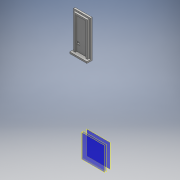
# Autodesk Inventor part: goraczesc1zotworem
Saved by Autodesk Inventor 2016 SP1 (Build 200210100, 210)
## iProperties
Created: 2019-02-21
Part Number: goraczesc1zotworem
Material: Ogólny
Document SubType Name: Modeling
Designer: Maciek
Density: 1 g/cm^3
Appearance: Domyślna
Author: Maciek
Autodesk Inventor part; units mm, degrees
ref_plane "YZ Plane" through (0, 0, 0) normal (1, 0, 0) x (0, 1, 0)
ref_plane "XZ Plane" through (0, 0, 0) normal (0, 1, 0) x (-1, 0, 0)
ref_plane "XY Plane" through (0, 0, 0) normal (0, 0, 1) x (1, 0, 0)
ref_plane "Płaszczyzna konstrukcyjna1" through (0, 19, 0) normal (0, 1, 0) x (1, 0, 0)
ref_plane "Płaszczyzna konstrukcyjna3" through (0, 19, 0) normal (0, 1, 0) x (1, 0, 0)
ref_plane "Płaszczyzna konstrukcyjna2" through (0, 24, 0) normal (0, 1, 0) x (1, 0, 0)
sketch "Szkic23" plane through (0, 24, 0) normal (0, 1, 0) x (1, 0, 0)
  line L0 (-21.8, -101.1) -> (-21.8, -97.6) projected
  line L1 (-8.8, -67.6) -> (-8.8, -69.1) projected
  line L2 (-21.8, -101.1) -> (-8.8, -101.1)
  line L3 (-8.8, -101.1) -> (-8.8, -69.1)
  line L4 (-8.8, -69.1) -> (-21.8, -69.1)
  line L5 (-21.8, -69.1) -> (-21.8, -101.1)
  line L6 (-21.8, -101.1) -> (-20.3, -101.1) construction
  line L7 (-20.3, -101.1) -> (-20.3, -99.6) construction
  line L8 (-20.3, -99.6) -> (-21.8, -99.6) construction
  line L9 (-21.8, -99.6) -> (-21.8, -101.1) construction
  line L10 (-8.8, -69.1) -> (-10.3, -69.1) construction
  line L11 (-21.8, -69.1) -> (-8.8, -69.1) construction
  line L12 (-20.3, -99.6) -> (-10.3, -99.6)
  line L13 (-10.3, -99.6) -> (-10.3, -69.1)
  line L14 (-10.3, -69.1) -> (-20.3, -69.1)
  line L15 (-20.3, -69.1) -> (-20.3, -99.6)
  point P0 (0, 0)
  dimension "d135" = 1.5
  dimension "d136" = 1.5
  dimension "d137" = 1.5
  constraints: 26 end point, 6 parallel, 3 horizontal, 3 perpendicular, 1 point on line
  measures "d135" distance of L8.end L7.end
  measures "d136" distance of L7.end L6.end
  measures "d137" distance of L1.end L10.end
extrude "Wyciągnięcie proste21" add sketch "Szkic23" against normal blind 1.5 contours L0 L5 L4 L15 L12 L13 L3 L2
ref_plane "Płaszczyzna konstrukcyjna5" through (0, 24, 0) normal (0, 1, 0) x (1, 0, 0)
sketch "Szkic24" plane through (0, 24, 0) normal (0, 1, 0) x (1, 0, 0)
  line L0 (-23.3, -69.1) -> (-23.3, -102.6) projected
  line L1 (-23.3, -69.1) -> (-7.3, -69.1)
  line L2 (-7.3, -69.1) -> (-7.3, -67.6)
  line L3 (-7.3, -67.6) -> (-23.3, -67.6)
  line L4 (-23.3, -67.6) -> (-23.3, -69.1)
  point P0 (0, 0)
  dimension "d140" = 16
  dimension "d141" = 1.5
  constraints: 8 end point, 2 parallel, 1 horizontal, 1 perpendicular
  measures "d140" distance of L3.end L2.end
  measures "d141" distance of L2.end L1.end
extrude "Wyciągnięcie proste22" add sketch "Szkic24" against normal blind 3.5
ref_plane "Płaszczyzna konstrukcyjna6" through (0, 24, 0) normal (0, 1, 0) x (1, 0, 0)
sketch "Szkic25" plane through (0, 24, 0) normal (0, 1, 0) x (1, 0, 0)
  line L0 (-7.3, -102.6) -> (-7.3, -69.1) projected
  line L1 (-23.3, -69.1) -> (-23.3, -67.6) projected
  line L2 (-7.3, -102.6) -> (-23.3, -102.6)
  line L3 (-23.3, -102.6) -> (-23.3, -67.6)
  line L4 (-23.3, -67.6) -> (-7.3, -67.6)
  line L5 (-7.3, -67.6) -> (-7.3, -102.6)
  point P0 (0, 0)
  constraints: 8 end point, 2 parallel, 1 horizontal, 1 perpendicular
extrude "Wyciągnięcie proste23" add sketch "Szkic25" along normal blind 1.5
ref_plane "Płaszczyzna konstrukcyjna4" through (0, 20.5, 0) normal (0, 1, 0) x (1, 0, 0)
sketch "Szkic27" plane through (0, 25.5, 0) normal (0, 1, 0) x (1, 0, 0)
  line L0 (-23.3, -67.6) -> (-23.3, -102.6) construction
  line L1 (-23.3, -102.6) -> (-23.3, -77.6) construction
  line L2 (-23.3, -77.6) -> (-23.3, -75.6) construction
  line L3 (-23.3, -77.6) -> (-20.3, -77.6) construction
  line L4 (-23.3, -75.6) -> (-17.3, -75.6) construction
  line L5 (-20.3, -77.6) -> (-17.3, -77.6)
  line L6 (-17.3, -77.6) -> (-17.3, -75.6)
  line L7 (-17.3, -75.6) -> (-20.3, -75.6)
  line L8 (-20.3, -75.6) -> (-20.3, -77.6)
  point P0 (0, 0)
  dimension "d152" = 25
  dimension "d153" = 2
  dimension "d154" = 3
  dimension "d155" = 6
  constraints: 16 end point, 2 horizontal, 2 parallel, 2 perpendicular, 2 point on line
  measures "d152" distance of L0.end L1.end
  measures "d153" distance of L1.end L2.end
  measures "d154" distance of L1.end L3.end
  measures "d155" distance of L2.end L4.end
extrude "Wyciągnięcie proste25" cut sketch "Szkic27" against normal blind 10
